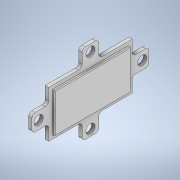
# Autodesk Inventor part: gehaeuse_deckel
Saved by Autodesk Inventor 2020 (Build 240168000, 168)
## iProperties
Created: 2020-05-23
Part Number: gehaeuse_deckel
Material: Generisch
Document SubType Name: Modeling
Designer: chris
Density: 1 g/cm^3
Appearance: Vorgabe
Author: chris
Autodesk Inventor part; units mm, degrees
ref_plane "YZ Plane" through (0, 0, 0) normal (1, 0, 0) x (0, 1, 0)
ref_plane "XZ Plane" through (0, 0, 0) normal (0, 1, 0) x (-1, 0, 0)
ref_plane "XY Plane" through (0, 0, 0) normal (0, 0, 1) x (1, 0, 0)
sketch "Skizze1" plane through (0, 0, 0) normal (1, 0, 0) x (0, 1, 0)
  line L0 (0, 0) -> (28, 0)
  line L1 (28, 0) -> (28, -50)
  line L2 (28, -50) -> (0, -50)
  line L3 (0, -50) -> (0, 0)
  dimension "d0" = 50
  dimension "d1" = 28
  constraints: 8 end point, 2 parallel, 1 horizontal, 1 perpendicular
  measures "d0" distance of L2.end L0.start
  measures "d1" distance of L0.start L0.end
extrude "Extrusion1" add sketch "Skizze1" along normal blind 2
sketch "Skizze2" plane through (2, 0, 0) normal (1, 0, 0) x (0, 0, -1)
  line L0 (2.2, 25.8) -> (47.8, 25.8)
  line L1 (47.8, 25.8) -> (47.8, 2.2)
  line L2 (47.8, 2.2) -> (2.2, 2.2)
  line L3 (2.2, 2.2) -> (2.2, 25.8)
  line L4 (0, 28) -> (0, 0) projected
  line L5 (0, 0) -> (50, 0) projected
  dimension "d4" = 45.6
  dimension "d5" = 23.6
  dimension "d6" = 2.2
  dimension "d7" = 2.2
  constraints: 8 end point, 2 parallel, 1 horizontal, 1 perpendicular
  measures "d4" distance between parallel lines of L1 L3
  measures "d5" distance between parallel lines of L2 L0
  measures "d6" distance between parallel lines of L4 L3
  measures "d7" distance between parallel lines of L5 L2
extrude "Extrusion2" add sketch "Skizze2" along normal blind 1.5
chamfer "Fase1" distance 0.5 angle 45 4 edges at (3.5, 2.2, -25) (3.5, 14, -2.2) (3.5, 14, -47.8) (3.5, 25.8, -25)
sketch "Skizze3" plane through (0, 0, 0) normal (-1, 0, 0) x (0, 0, 1)
  line L0 (-50, 0) -> (-50, 28) projected
  line L1 (-50, 9) -> (-60, 9)
  line L2 (-60, 9) -> (-60, 19)
  line L3 (-60, 19) -> (-50, 19)
  line L4 (-50, 19) -> (-50, 9)
  line L5 (-50, 28) -> (0, 28) projected
  line L6 (-30, 28) -> (-20, 28)
  line L7 (-20, 28) -> (-20, 38)
  line L8 (-20, 38) -> (-30, 38)
  line L9 (-30, 38) -> (-30, 28)
  line L10 (-30, 0) -> (-20, 0)
  line L11 (-20, 0) -> (-20, -10)
  line L12 (-20, -10) -> (-30, -10)
  line L13 (-30, -10) -> (-30, 0)
  line L14 (0, 28) -> (0, 0) projected
  line L15 (0, 9) -> (10, 9)
  line L16 (10, 9) -> (10, 19)
  line L17 (10, 19) -> (0, 19)
  line L18 (0, 19) -> (0, 9)
  line L19 (0, 0) -> (-50, 0) projected
  point P0 (0, 19)
  dimension "d13" = 10
  dimension "d14" = 10
  dimension "d15" = 10
  dimension "d16" = 10
  dimension "d17" = 10
  dimension "d18" = 10
  dimension "d19" = 10
  dimension "d20" = 10
  dimension "d21" = 20
  dimension "d22" = 20
  dimension "d23" = 9
  dimension "d24" = 9
  constraints: 32 end point, 8 parallel, 4 horizontal, 4 perpendicular, 3 point on line, 1 collinear
  measures "d13" distance between parallel lines of L3 L1
  measures "d14" distance between parallel lines of L7 L9
  measures "d15" distance between parallel lines of L17 L15
  measures "d16" distance between parallel lines of L11 L13
  measures "d17" distance between parallel lines of L0 L2
  measures "d18" distance between parallel lines of L5 L8
  measures "d19" distance between parallel lines of L16 L18
  measures "d20" distance between parallel lines of L10 L12
  measures "d21" distance between parallel lines of L14 L11
  measures "d22" distance between parallel lines of L14 L7
  measures "d23" distance between parallel lines of L19 L15
  measures "d24" distance between parallel lines of L19 L1
extrude "Extrusion3" add sketch "Skizze3" against normal blind 2 contours L1 L2 L3 L0 | L10 L11 L12 L13 | L9 L8 L7 L5 | L14 L17 L16 L15
fillet "Rundung1" radius 2 16 edges at (1, 28, -30) (1, 38, -30) (1, 38, -20) (1, 19, -50) (1, 19, -60) (1, 9, -60) (1, 19, 10) (1, -10, -30) (1, 9, -50) (1, -10, -20) (1, 9, 10) (1, 0, -20) (1, 9, 0) (1, 19, 0) (1, 28, -20) (1, 0, -30)
sketch "Skizze4" plane through (0, 0, 0) normal (-1, 0, 0) x (0, 0, 1)
  circle A0 centre (-25, 34) radius 2.75
  circle A1 centre (6, 14) radius 2.75
  circle A2 centre (-25, -6) radius 2.75
  circle A3 centre (-56, 14) radius 2.75
  line L0 (-30, 36) -> (-30, 30) projected
  line L1 (-52, 19) -> (-58, 19) projected
  line L2 (8, 19) -> (2, 19) projected
  line L3 (-30, -2) -> (-30, -8) projected
  line L4 (10, 11) -> (10, 17) projected
  line L5 (-28, -10) -> (-22, -10) projected
  line L6 (-60, 17) -> (-60, 11) projected
  line L7 (-22, 38) -> (-28, 38) projected
  point P0 (0, 0)
  dimension "d28" = 5.5
  dimension "d29" = 5
  dimension "d30" = 5
  dimension "d31" = 5
  dimension "d32" = 5
  dimension "d33" = 4
  dimension "d34" = 4
  dimension "d35" = 4
  dimension "d36" = 4
  constraints: 4 centre point, 3 equal radius
  measures "d28" diameter of A0
  measures "d29" distance from line of L0 A0.centre
  measures "d30" distance from line of L1 A3.centre
  measures "d31" distance from line of L2 A1.centre
  measures "d32" distance from line of L3 A2.centre
  measures "d33" distance from line of L4 A1.centre
  measures "d34" distance from line of A2.centre L5
  measures "d35" distance from line of A3.centre L6
  measures "d36" distance from line of L7 A0.centre
extrude "Extrusion4" cut sketch "Skizze4" against normal blind 2
